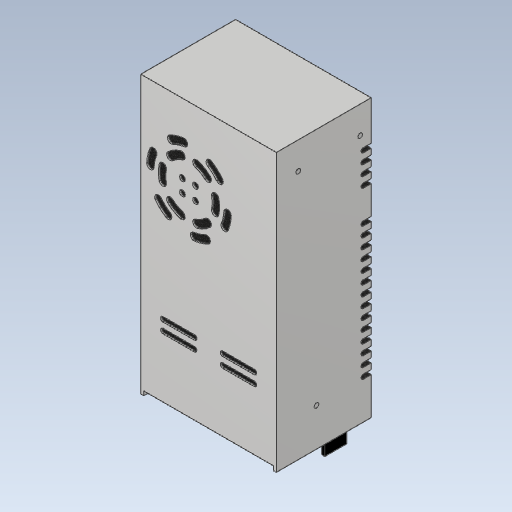
# Autodesk Inventor part: Meanwell S-240-24 24V 10A PSU
Saved by Autodesk Inventor 2020 (Build 240168000, 168)
## iProperties
Created: 2018-11-04
Part Number: Meanwell S-240-24 24V 10A PSU
Material: Aluminum 5454 0 Cold Formed
Document SubType Name: Modeling
Designer: LillaHunden
Density: 2.69 g/cm^3
Appearance: Satin
Mass: 3032.72 g
Surface Area: 850.483 cm^2
Volume: 1127.4 cm^3
Author: LillaHunden
Autodesk Inventor part; units mm, degrees
ref_plane "YZ Plane" through (0, 0, 0) normal (1, 0, 0) x (0, 1, 0)
ref_plane "XZ Plane" through (0, 0, 0) normal (0, 1, 0) x (-1, 0, 0)
sketch "Sketch1" plane through (0, 0, 0) normal (1, 0, 0) x (0, 1, 0)
  line L0 (-95, -32.5) -> (95, -32.5)
  line L1 (95, -32.5) -> (95, 32.5)
  line L2 (95, 32.5) -> (-95, 32.5)
  line L3 (-95, 32.5) -> (-95, -32.5)
  line L4 (-95, -32.5) -> (95, 32.5) construction
  line L5 (95, -32.5) -> (-95, 32.5) construction
  point P0 (0, 0)
  dimension "d0" = 190
  dimension "d1" = 65
  constraints: 12 end point, 2 midpoint, 2 parallel, 1 horizontal, 1 perpendicular
  measures "d0" distance of L2.end L1.end
  measures "d1" distance of L1.end L0.end
extrude "Extrusion1" add sketch "Sketch1" along normal blind 93
sketch "Sketch3" plane through (93, 0, 0) normal (1, 0, 0) x (0, 0, -1)
  line L0 (32.5, -95) -> (32.5, 95) projected
  line L1 (-32.5, -95) -> (32.5, -95) projected
  point P0 (0, 0)
  point P1 (-5, -69)
  point P2 (-17.5, 76.25)
  point P3 (25, 76.25)
  dimension "d8" = 37.5
  dimension "d9" = 26
  dimension "d10" = 7.5
  dimension "d11" = 50
  dimension "d12" = 171.25
  constraints: 1 horizontal alignment
  measures "d8" distance from line of L0 point (-5, -69)
  measures "d9" distance from line of L1 point (-5, -69)
  measures "d10" distance from line of L0 point (25, 76.25)
  measures "d11" distance from line of L0 point (-17.5, 76.25)
  measures "d12" distance from line of L1 point (-17.5, 76.25)
hole "Hole1" at (93, -69, 5) at (93, 76.25, 17.5) at (93, 76.25, -25) direction (-1, 0, 0) diameter 3.242 depth 11.8 tip angle 118 thread size "M4x0.7" class "6H" standard "ISO Metric profile"
sketch "Sketch4" plane through (0, -95, 32.5) normal (0, 0, 1) x (1, 0, 0)
  line L0 (0, 0) -> (93, 0) projected
  line L1 (93, 190) -> (93, 0) projected
  circle A0 centre (28.5, 133.5) radius 2
  circle A1 centre (28.5, 142.5) radius 2
  circle A2 centre (37.5, 142.5) radius 2
  circle A3 centre (37.5, 133.5) radius 2
  line L2 (28.5, 133.5) -> (28.5, 142.5) construction
  line L3 (28.5, 142.5) -> (37.5, 142.5) construction
  line L4 (37.5, 142.5) -> (37.5, 133.5) construction
  line L5 (39.5, 132.1703) -> (39.5, 138.3167) construction
  line L6 (26.5, 133.1483) -> (26.5, 137.8908) construction
  line L7 (25.9466, 144.5) -> (41.2052, 144.5) construction
  line L8 (25.4076, 131.5) -> (44.4725, 131.5) construction
  line L9 (37.5, 133.5) -> (28.5, 133.5) construction
  point P0 (0, 95)
  point P1 (33, 138)
  point P2 (28.5, 138)
  point P3 (33, 135.1483)
  point P4 (33, 133.5)
  dimension "d20" = 138
  dimension "d21" = 60
  dimension "d22" = 4
  dimension "d23" = 4
  dimension "d24" = 4
  dimension "d25" = 4
  dimension "d26" = 13
  dimension "d27" = 13
  constraints: 16 end point, 4 centre point, 4 tangent, 4 vertical alignment, 3 horizontal, 3 horizontal alignment, 3 vertical, 2 midpoint, 2 perpendicular
  measures "d20" distance from line of L0 point (33, 138)
  measures "d21" distance from line of L1 point (33, 138)
  measures "d22" diameter of A0
  measures "d23" diameter of A3
  measures "d24" diameter of A2
  measures "d25" diameter of A1
  measures "d26" distance between parallel lines of L6 L5
  measures "d27" distance between parallel lines of L7 L8
extrude "Extrusion2" cut sketch "Sketch4" against normal blind 1
sketch "Sketch5" plane through (0, -95, 32.5) normal (0, 0, 1) x (1, 0, 0)
  circle A0 centre (28.5, 133.5) radius 2 projected
  circle A1 centre (28.5, 142.5) radius 2 projected
  circle A2 centre (37.5, 142.5) radius 2 projected
  circle A3 centre (37.5, 133.5) radius 2 projected
  circle A4 centre (28.5, 133.5) radius 2 construction
  line L0 (28.5, 133.5) -> (37.5, 142.5) construction
  line L1 (37.5, 142.5) -> (37.5, 133.5) construction
  circle A5 centre (28.5, 142.5) radius 2 construction
  line L2 (37.5, 133.5) -> (28.5, 142.5) construction
  circle A6 centre (33, 138) radius 29 construction
  circle A7 centre (33, 138) radius 24 construction
  arc A8 (8.5172, 148.1411) -> (6.5252, 139.1559) centre (33, 138) ccw construction
  arc A9 (6.2075, 149.0978) -> (4.0276, 139.265) centre (33, 138) ccw
  arc A10 (10.8269, 147.1844) -> (9.0228, 139.0469) centre (33, 138) ccw
  arc A11 (10.8269, 147.1844) -> (6.2075, 149.0978) centre (8.5172, 148.1411) ccw
  arc A12 (4.0276, 139.265) -> (9.0228, 139.0469) centre (6.5252, 139.1559) ccw
  line L3 (33, 138) -> (6.5252, 139.1559) construction
  line L4 (33, 138) -> (59.5, 138) construction
  line L5 (33, 138) -> (8.5172, 148.1411) construction
  arc A13 (17.4183, 113.5416) -> (20.1048, 117.7586) centre (18.7616, 115.6501) ccw
  arc A14 (13.9595, 123.3897) -> (20.1048, 117.7586) centre (33, 138) ccw
  arc A15 (11.9761, 121.8678) -> (18.7616, 115.6501) centre (33, 138) ccw construction
  arc A16 (13.9595, 123.3897) -> (9.9928, 120.3459) centre (11.9761, 121.8678) ccw
  arc A17 (9.9928, 120.3459) -> (17.4183, 113.5416) centre (33, 138) ccw
  arc A18 (46.3907, 112.2767) -> (44.082, 116.7117) centre (45.2363, 114.4942) ccw
  arc A19 (36.1326, 114.2053) -> (44.082, 116.7117) centre (33, 138) ccw
  arc A20 (36.4589, 111.7267) -> (45.2363, 114.4942) centre (33, 138) ccw construction
  arc A21 (36.1326, 114.2053) -> (36.7853, 109.2481) centre (36.4589, 111.7267) ccw
  arc A22 (36.7853, 109.2481) -> (46.3907, 112.2767) centre (33, 138) ccw
  arc A23 (61.9724, 136.735) -> (56.9772, 136.9531) centre (59.4748, 136.8441) ccw
  arc A24 (55.1731, 128.8156) -> (56.9772, 136.9531) centre (33, 138) ccw
  arc A25 (57.4828, 127.8589) -> (59.4748, 136.8441) centre (33, 138) ccw construction
  arc A26 (55.1731, 128.8156) -> (59.7925, 126.9022) centre (57.4828, 127.8589) ccw
  arc A27 (59.7925, 126.9022) -> (61.9724, 136.735) centre (33, 138) ccw
  arc A28 (48.5817, 162.4584) -> (45.8952, 158.2414) centre (47.2384, 160.3499) ccw
  arc A29 (52.0405, 152.6103) -> (45.8952, 158.2414) centre (33, 138) ccw
  arc A30 (54.0239, 154.1322) -> (47.2384, 160.3499) centre (33, 138) ccw construction
  arc A31 (52.0405, 152.6103) -> (56.0072, 155.6541) centre (54.0239, 154.1322) ccw
  arc A32 (56.0072, 155.6541) -> (48.5817, 162.4584) centre (33, 138) ccw
  arc A33 (19.6093, 163.7233) -> (21.918, 159.2883) centre (20.7637, 161.5058) ccw
  arc A34 (29.8674, 161.7947) -> (21.918, 159.2883) centre (33, 138) ccw
  arc A35 (29.5411, 164.2733) -> (20.7637, 161.5058) centre (33, 138) ccw construction
  arc A36 (29.8674, 161.7947) -> (29.2147, 166.7519) centre (29.5411, 164.2733) ccw
  arc A37 (29.2147, 166.7519) -> (19.6093, 163.7233) centre (33, 138) ccw
  point P0 (0, 95)
  dimension "d30" = 58
  dimension "d31" = 48
  dimension "d32" = 26.5
  dimension "d33" = 177.5
  dimension "d34" = 20
  dimension "d35" = 5
  dimension "d36" = 14.2034
  dimension "d39" = 360
  constraints: 60 point on circle, 32 centre point, 12 end point, 4 tangent, 3 coincident, 1 concentric, 1 equal length, 1 horizontal, 1 midpoint, 1 perpendicular, 1 vertical, 73 other
  measures "d30" diameter of A6
  measures "d31" diameter of A7
  measures "d32" radius of A8
  measures "d33" angle of L4 L3
  measures "d34" angle of L5 L3
  measures "d35" diameter of A11
extrude "Extrusion3" cut sketch "Sketch5" against normal blind 1 contours A11 A10 A12 A9 | A17 A16 A14 A13 | A22 A21 A19 A18 | A27 A26 A24 A23 | A32 A31 A29 A28 | A37 A36 A34 A33
sketch "Sketch6" plane through (0, -95, 32.5) normal (0, 0, 1) x (1, 0, 0)
  circle A0 centre (28.5, 133.5) radius 2 construction
  circle A1 centre (37.5, 142.5) radius 2 construction
  line L0 (28.5, 133.5) -> (37.5, 142.5) construction
  circle A2 centre (37.5, 133.5) radius 2 construction
  circle A3 centre (28.5, 142.5) radius 2 construction
  line L1 (37.5, 133.5) -> (28.5, 142.5) construction
  arc A4 (17.4793, 141.8868) -> (17.4793, 134.1132) centre (33, 138) ccw
  arc A5 (15.0542, 142.4941) -> (14.5, 138) centre (33, 138) ccw construction
  arc A6 (12.629, 143.1014) -> (12, 138) centre (33, 138) ccw
  arc A7 (17.4793, 141.8868) -> (17, 138) centre (33, 138) ccw
  arc A8 (17.4793, 141.8868) -> (12.629, 143.1014) centre (15.0542, 142.4941) ccw
  arc A9 (12, 138) -> (17, 138) centre (14.5, 138) ccw construction
  line L2 (12, 138) -> (17, 138) construction
  arc A10 (12.629, 132.8986) -> (17.4793, 134.1132) centre (15.0542, 133.5059) ccw
  arc A11 (12, 138) -> (12.629, 132.8986) centre (33, 138) ccw
  arc A12 (22.5, 119.8135) -> (25, 124.1436) centre (23.75, 121.9785) ccw construction
  arc A13 (22.5, 119.8135) -> (27.2324, 117.8075) centre (33, 138) ccw
  line L3 (22.5, 119.8135) -> (25, 124.1436) construction
  arc A14 (27.2324, 117.8075) -> (28.6057, 122.6153) centre (27.9191, 120.2114) ccw
  arc A15 (20.1351, 124.7055) -> (23.75, 121.9785) centre (33, 138) ccw construction
  arc A16 (18.3966, 122.9089) -> (22.5, 119.8135) centre (33, 138) ccw
  arc A17 (21.8736, 126.502) -> (18.3966, 122.9089) centre (20.1351, 124.7055) ccw
  arc A18 (21.8736, 126.502) -> (28.6057, 122.6153) centre (33, 138) ccw
  arc A19 (21.8736, 126.502) -> (25, 124.1436) centre (33, 138) ccw
  arc A20 (43.5, 119.8135) -> (41, 124.1436) centre (42.25, 121.9785) ccw construction
  arc A21 (43.5, 119.8135) -> (47.6034, 122.9089) centre (33, 138) ccw
  line L4 (43.5, 119.8135) -> (41, 124.1436) construction
  arc A22 (47.6034, 122.9089) -> (44.1264, 126.502) centre (45.8649, 124.7055) ccw
  arc A23 (38.0809, 120.2114) -> (42.25, 121.9785) centre (33, 138) ccw construction
  arc A24 (38.7676, 117.8075) -> (43.5, 119.8135) centre (33, 138) ccw
  arc A25 (37.3943, 122.6153) -> (38.7676, 117.8075) centre (38.0809, 120.2114) ccw
  arc A26 (37.3943, 122.6153) -> (44.1264, 126.502) centre (33, 138) ccw
  arc A27 (37.3943, 122.6153) -> (41, 124.1436) centre (33, 138) ccw
  arc A28 (54, 138) -> (49, 138) centre (51.5, 138) ccw construction
  arc A29 (54, 138) -> (53.371, 143.1014) centre (33, 138) ccw
  line L5 (54, 138) -> (49, 138) construction
  arc A30 (53.371, 143.1014) -> (48.5207, 141.8868) centre (50.9458, 142.4941) ccw
  arc A31 (50.9458, 133.5059) -> (51.5, 138) centre (33, 138) ccw construction
  arc A32 (53.371, 132.8986) -> (54, 138) centre (33, 138) ccw
  arc A33 (48.5207, 134.1132) -> (53.371, 132.8986) centre (50.9458, 133.5059) ccw
  arc A34 (48.5207, 134.1132) -> (48.5207, 141.8868) centre (33, 138) ccw
  arc A35 (48.5207, 134.1132) -> (49, 138) centre (33, 138) ccw
  arc A36 (43.5, 156.1865) -> (41, 151.8564) centre (42.25, 154.0215) ccw construction
  arc A37 (43.5, 156.1865) -> (38.7676, 158.1925) centre (33, 138) ccw
  line L6 (43.5, 156.1865) -> (41, 151.8564) construction
  arc A38 (38.7676, 158.1925) -> (37.3943, 153.3847) centre (38.0809, 155.7886) ccw
  arc A39 (45.8649, 151.2945) -> (42.25, 154.0215) centre (33, 138) ccw construction
  arc A40 (47.6034, 153.0911) -> (43.5, 156.1865) centre (33, 138) ccw
  arc A41 (44.1264, 149.498) -> (47.6034, 153.0911) centre (45.8649, 151.2945) ccw
  arc A42 (44.1264, 149.498) -> (37.3943, 153.3847) centre (33, 138) ccw
  arc A43 (44.1264, 149.498) -> (41, 151.8564) centre (33, 138) ccw
  arc A44 (22.5, 156.1865) -> (25, 151.8564) centre (23.75, 154.0215) ccw construction
  arc A45 (22.5, 156.1865) -> (18.3966, 153.0911) centre (33, 138) ccw
  line L7 (22.5, 156.1865) -> (25, 151.8564) construction
  arc A46 (18.3966, 153.0911) -> (21.8736, 149.498) centre (20.1351, 151.2945) ccw
  arc A47 (27.9191, 155.7886) -> (23.75, 154.0215) centre (33, 138) ccw construction
  arc A48 (27.2324, 158.1925) -> (22.5, 156.1865) centre (33, 138) ccw
  arc A49 (28.6057, 153.3847) -> (27.2324, 158.1925) centre (27.9191, 155.7886) ccw
  arc A50 (28.6057, 153.3847) -> (21.8736, 149.498) centre (33, 138) ccw
  arc A51 (28.6057, 153.3847) -> (25, 151.8564) centre (33, 138) ccw
  point P0 (0, 95)
  dimension "d43" = 32
  dimension "d46" = 5
  dimension "d49" = 360
  constraints: 96 point on circle, 48 centre point, 16 end point, 5 tangent, 3 coincident, 3 symmetric about line, 1 horizontal, 1 midpoint, 126 other
  measures "d43" diameter of A4
  measures "d46" diameter of A8
extrude "Extrusion4" cut sketch "Sketch6" against normal blind 1
sketch "Sketch7" plane through (0, -95, 32.5) normal (0, 0, 1) x (1, 0, 0)
  line L0 (13.5, 52) -> (79.5, 52) construction
  line L1 (13.5, 45) -> (79.5, 45) construction
  line L2 (93, 190) -> (93, 0) construction
  line L3 (0, 0) -> (93, 0) construction
  line L4 (13.5, 52) -> (38.5, 52) construction
  line L5 (15.1, 50.4) -> (36.9, 50.4)
  line L6 (36.9, 53.6) -> (15.1, 53.6)
  arc A0 (15.1, 53.6) -> (15.1, 50.4) centre (15.1, 52) ccw
  arc A1 (36.9, 50.4) -> (36.9, 53.6) centre (36.9, 52) ccw
  line L7 (13.5, 52) -> (38.5, 52) construction
  line L8 (79.5, 52) -> (54.5, 52) construction
  line L9 (77.9, 53.6) -> (56.1, 53.6)
  line L10 (56.1, 50.4) -> (77.9, 50.4)
  arc A2 (77.9, 50.4) -> (77.9, 53.6) centre (77.9, 52) ccw
  arc A3 (56.1, 53.6) -> (56.1, 50.4) centre (56.1, 52) ccw
  line L11 (79.5, 45) -> (54.5, 45) construction
  line L12 (77.9, 46.6) -> (56.1, 46.6)
  line L13 (56.1, 43.4) -> (77.9, 43.4)
  arc A4 (77.9, 43.4) -> (77.9, 46.6) centre (77.9, 45) ccw
  arc A5 (56.1, 46.6) -> (56.1, 43.4) centre (56.1, 45) ccw
  line L14 (13.5, 45) -> (38.5, 45) construction
  line L15 (15.1, 46.6) -> (36.9, 46.6)
  line L16 (36.9, 43.4) -> (15.1, 43.4)
  arc A6 (15.1, 46.6) -> (15.1, 43.4) centre (15.1, 45) ccw
  arc A7 (36.9, 43.4) -> (36.9, 46.6) centre (36.9, 45) ccw
  point P0 (0, 95)
  point P1 (26, 52)
  point P2 (67, 52)
  point P3 (67, 45)
  point P4 (26, 45)
  dimension "d53" = 66
  dimension "d54" = 13.5
  dimension "d55" = 7
  dimension "d56" = 52
  dimension "d57" = 25
  dimension "d58" = 0
  dimension "d59" = 3.2
  dimension "d60" = 25
  dimension "d61" = 3.2
  dimension "d62" = 3.2
  constraints: 38 end point, 24 point on circle, 16 tangent, 11 point on line, 8 centre point, 4 midpoint, 4 parallel, 3 horizontal, 2 collinear, 2 vertical alignment
  measures "d53" distance of L0.start L0.end
  measures "d54" distance from line of L2 L0.end
  measures "d55" distance of L1.start L0.start
  measures "d56" distance from line of L3 L0.end
  measures "d57" distance of L0.start L4.end
  measures "d58" distance between parallel lines of L4 L7
  measures "d59" diameter of A1
  measures "d60" distance of L0.end L8.end
  measures "d61" diameter of A3
  measures "d62" diameter of A5
extrude "Extrusion5" cut sketch "Sketch7" against normal blind 1
sketch "Sketch8" plane through (0, -95, -32.5) normal (0, -1, 0) x (1, 0, 0)
  line L0 (19.2, 27) -> (88.2, 27)
  line L1 (88.2, 27) -> (88.2, 12)
  line L2 (88.2, 12) -> (19.2, 12)
  line L3 (19.2, 12) -> (19.2, 27)
  line L4 (93, 65) -> (93, 0) projected
  line L5 (0, 0) -> (93, 0) projected
  point P0 (0, 32.5)
  dimension "d65" = 4.8
  dimension "d66" = 69
  dimension "d67" = 15
  dimension "d68" = 12
  constraints: 8 end point, 2 parallel, 1 horizontal, 1 perpendicular
  measures "d65" distance between parallel lines of L4 L1
  measures "d66" distance of L0.start L0.end
  measures "d67" distance of L2.end L0.start
  measures "d68" distance between parallel lines of L5 L2
extrude "Extrusion6" add sketch "Sketch8" along normal blind 12
sketch "Sketch9" plane through (0, -95, -32.5) normal (0, -1, 0) x (1, 0, 0)
  line L0 (91, 65) -> (2, 65)
  line L1 (2, 65) -> (2, 27)
  line L2 (2, 27) -> (91, 27)
  line L3 (91, 27) -> (91, 65)
  line L4 (36.9, 65) -> (38.5, 65) projected
  line L5 (0, 65) -> (0, 0) projected
  line L6 (93, 65) -> (93, 0) projected
  line L7 (88.2, 27) -> (19.2, 27) projected
  point P0 (0, 32.5)
  point P1 (37.7, 65)
  point P2 (46.5, 27)
  dimension "d71" = 2
  dimension "d72" = 2
  constraints: 8 end point, 2 midpoint, 2 parallel, 2 point on line, 1 horizontal, 1 perpendicular
  measures "d71" distance between parallel lines of L5 L1
  measures "d72" distance between parallel lines of L6 L3
extrude "Extrusion7" cut sketch "Sketch9" against normal blind 2.85
sketch "Sketch10" plane through (0, -95, -32.5) normal (0, -1, 0) x (1, 0, 0)
  line L0 (19.2, 27) -> (2, 27) projected
  line L1 (19.2, 27) -> (2, 27)
  line L2 (2, 27) -> (2, 12)
  line L3 (2, 12) -> (19.2, 12)
  line L4 (19.2, 12) -> (19.2, 27)
  point P0 (0, 32.5)
  constraints: 8 end point, 2 parallel, 1 horizontal, 1 perpendicular
extrude "Extrusion8" cut sketch "Sketch10" against normal up to surface (2.85 mm away)
sketch "Sketch11" plane through (0, 0, 0) normal (-1, 0, 0) x (0, 0, 1)
  line L0 (17, -87.5) -> (-8, -87.5) construction
  line L1 (15.5, -86) -> (-6.5, -86)
  line L2 (-6.5, -89) -> (15.5, -89)
  arc A0 (15.5, -89) -> (15.5, -86) centre (15.5, -87.5) ccw
  arc A1 (-6.5, -86) -> (-6.5, -89) centre (-6.5, -87.5) ccw
  line L3 (32.5, -95) -> (-32.5, -95) projected
  line L4 (32.5, 95) -> (32.5, -95) projected
  point P0 (0, 0)
  point P1 (4.5, -87.5)
  dimension "d77" = 25
  dimension "d78" = 3
  dimension "d79" = 6
  dimension "d80" = 15.5
  constraints: 8 end point, 6 point on circle, 4 tangent, 2 centre point, 2 point on line, 1 horizontal, 1 midpoint, 1 parallel
  measures "d77" distance of L0.start L0.end
  measures "d78" diameter of A1
  measures "d79" distance between parallel lines of L3 L2
  measures "d80" distance from line of L4 L0.start
extrude "Extrusion9" cut sketch "Sketch11" against normal blind 1
pattern_linear "Rectangular Pattern1" count 5 spacing 7.5 along (0, 1, 0) of "Extrusion9"
sketch "Sketch12" plane through (0, -95, -32.5) normal (0, 0, -1) x (-1, 0, 0)
  line L0 (3.7427, 27) -> (-18, 27) construction
  line L1 (2.2427, 28.5) -> (-16.5, 28.5)
  line L2 (-16.5, 25.5) -> (2.2427, 25.5)
  arc A0 (2.2427, 25.5) -> (2.2427, 28.5) centre (2.2427, 27) ccw
  arc A1 (-16.5, 28.5) -> (-16.5, 25.5) centre (-16.5, 27) ccw
  line L3 (0, 0) -> (0, 190) projected
  line L4 (0, 0) -> (-93, 0) projected
  point P0 (0, 95)
  point P1 (-7.1287, 27)
  dimension "d86" = 3
  dimension "d87" = 18
  dimension "d94" = 27
  constraints: 8 end point, 6 point on circle, 4 tangent, 2 centre point, 2 point on line, 1 horizontal, 1 midpoint, 1 parallel
  measures "d86" diameter of A1
  measures "d87" distance from line of L3 L0.end
  measures "d94" distance from line of L4 L0.end
extrude "Extrusion10" cut sketch "Sketch12" against normal blind 7
fillet "Fillet1" radius 1.5 3 edges at (8.25, -66.5, -25.5) (18, -68, -25.5) (8.25, -69.5, -25.5)
pattern_linear "Rectangular Pattern2" count 14 spacing 7 along (0, 1, 0) of "Extrusion10", "Fillet1"
sketch "Sketch13" plane through (93, 95, -32.5) normal (0, 0, -1) x (-1, 0, 0)
  line L0 (95, -28.5) -> (75, -28.5) construction
  line L1 (93, -70.5) -> (93, 0) projected
  line L2 (93.5, -27) -> (76.5, -27)
  line L3 (76.5, -30) -> (93.5, -30)
  arc A0 (93.5, -30) -> (93.5, -27) centre (93.5, -28.5) ccw
  arc A1 (76.5, -27) -> (76.5, -30) centre (76.5, -28.5) ccw
  arc A2 (76.5, -70.5) -> (76.5, -73.5) centre (76.5, -72) ccw projected
  line L4 (93, 0) -> (0, 0) projected
  point P0 (93, -95)
  point P1 (85, -28.5)
  point P2 (75, -72)
  dimension "d95" = 3
  dimension "d96" = 20
  dimension "d97" = 27
  constraints: 8 end point, 7 point on circle, 4 tangent, 2 centre point, 2 point on line, 1 midpoint, 1 parallel, 1 perpendicular, 1 vertical alignment
  measures "d95" distance between parallel lines of L2 L3
  measures "d96" distance of L0.end L0.start
  measures "d97" distance between parallel lines of L4 L2
extrude "Extrusion11" cut sketch "Sketch13" against normal blind 7
fillet "Fillet2" radius 1.5 3 edges at (8.25, 65, -25.5) (18, 66.5, -25.5) (8.25, 68, -25.5)
pattern_linear "Rectangular Pattern3" count 4 spacing 7 along (0, -1, 0) of "Extrusion11", "Fillet2"
ref_plane "Work Plane1" through (46.5, 0, 0) normal (-1, 0, 0) x (0, 0, 1)
mirror "Mirror1" about plane through (46.5, 0, 0) normal (-1, 0, 0) of "Extrusion11", "Fillet2", "Rectangular Pattern3", "Extrusion10", "Fillet1", "Rectangular Pattern2"
sketch "Sketch14" plane through (19.2, -107, -5.5) normal (0, 0, 1) x (1, 0, 0)
  line L0 (2, 9.7) -> (10.2, 9.7)
  line L1 (10.2, 9.7) -> (10.2, 0)
  line L2 (10.2, 0) -> (2, 0)
  line L3 (2, 0) -> (2, 9.7)
  line L4 (0, 14.85) -> (0, 0) projected
  point P0 (-19.2, 107)
  dimension "d104" = 8.2
  dimension "d105" = 9.7
  dimension "d106" = 2
  constraints: 8 end point, 2 parallel, 1 horizontal, 1 perpendicular, 1 point on line
  measures "d104" distance of L1.end L2.end
  measures "d105" distance of L0.end L1.end
  measures "d106" distance between parallel lines of L4 L3
extrude "Extrusion12" cut sketch "Sketch14" against normal through all
pattern_linear "Rectangular Pattern4" count 7 spacing 9.45 along (1, 0, 0) of "Extrusion12"
hole "Hole2" at (25.3, -97.3, -13) direction (0, 1, 0) diameter 2.459 depth 8.8 tip angle 118 thread size "M3x0.5" class "6H" standard "ISO Metric profile"
hole "Hole3" at (34.75, -97.3, -13) direction (0, 1, 0) diameter 2.459 depth 8.8 tip angle 118 thread size "M3x0.5" class "6H" standard "ISO Metric profile"
hole "Hole4" at (44.2, -97.3, -13) direction (0, 1, 0) diameter 2.459 depth 8.8 tip angle 118 thread size "M3x0.5" class "6H" standard "ISO Metric profile"
hole "Hole5" at (53.65, -97.3, -13) direction (0, 1, 0) diameter 2.459 depth 8.8 tip angle 118 thread size "M3x0.5" class "6H" standard "ISO Metric profile"
hole "Hole6" at (63.1, -97.3, -13) direction (0, 1, 0) diameter 2.459 depth 8.8 tip angle 118 thread size "M3x0.5" class "6H" standard "ISO Metric profile"
hole "Hole7" at (82, -97.3, -13) direction (0, 1, 0) diameter 2.459 depth 8.8 tip angle 118 thread size "M3x0.5" class "6H" standard "ISO Metric profile"
hole "Hole8" at (72.55, -97.3, -13) direction (0, 1, 0) diameter 2.459 depth 8.8 tip angle 118 thread size "M3x0.5" class "6H" standard "ISO Metric profile"
equation "\"d23\" = d22"
equation "\"d24\" = d22"
equation "\"d25\" = d22"
equation "\"d72\" = d71"
body "Solid1"
